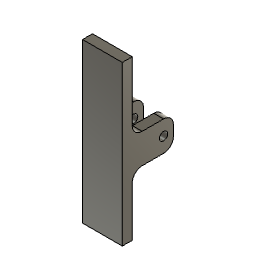
bending_tool_base v2 (Autodesk Fusion 360 design; units mm, degrees)
Autodesk Fusion 360 part; units mm, degrees
sketch "Skizze8" plane through (0, 0, 0) normal (1, 0, 0) x (0, 1, 0)
  line L0 (-6.5, 80) -> (-16.5, 80)
  line L1 (-16.5, 80) -> (-16.5, -80)
  line L2 (-16.5, -80) -> (-6.5, -80)
  line L3 (-6.5, -80) -> (-6.5, -30)
  line L4 (3.5, -20) -> (25, -20)
  line L5 (35, -10) -> (35, 0)
  line L6 (25, 10) -> (3.5, 10)
  line L7 (105.6778, -5) -> (-37.6639, -5) construction
  line L8 (25, 49.113) -> (25, -113.6091) construction
  line L9 (-6.5, 20) -> (-6.5, 80)
  arc A0 (-6.5, 20) -> (3.5, 10) centre (3.5, 20) ccw
  arc A1 (3.5, -20) -> (-6.5, -30) centre (3.5, -30) ccw
  arc A2 (35, 0) -> (25, 10) centre (25, 0) ccw
  arc A3 (25, -20) -> (35, -10) centre (25, -10) ccw
  circle A4 centre (25, -5) radius 4.15
  point P0 (-6.5, 10)
  dimension "d127" = 80
  dimension "d128" = 80
  dimension "d129" = 5
  dimension "d130" = 31.5
  dimension "d131" = 25
  dimension "d132" = 10
  dimension "d133" = 10
  dimension "d134" = 15
  dimension "d135" = 15
  dimension "d136" = 10
  dimension "d137" = 10
  dimension "d138" = 10
  dimension "d139" = 10
  dimension "d140" = 10
  dimension "d141" = 10
  dimension "d142" = 8.3
  constraint horizontal L0
  constraint perpendicular L0 L1
  constraint perpendicular L1 L2
  constraint perpendicular L2 L3
  constraint perpendicular L3 L4
  constraint perpendicular L4 L5
  constraint perpendicular L5 L6
  constraint perpendicular L1 L7
  constraint vertical L8
  constraint coincident P0 L6
  constraint coincident P0 L9
  constraint tangent L6 A0
  constraint tangent L9 A0
  constraint tangent L3 A1
  constraint tangent L4 A1
  constraint tangent L5 A2
  constraint tangent L6 A2
  constraint tangent L4 A3
  constraint tangent L5 A3
  constraint coincident L8 A4.centre
  constraint coincident L7 A4.centre
  measures "d127" distance of origin L0
  measures "d128" distance of origin L2
  measures "d129" distance of origin L7
  measures "d130" distance of L3 L8
  measures "d131" distance of origin L8
  measures "d132" distance of L1 L3
  measures "d133" distance of L5 L8
  measures "d134" distance of L4 L7
  measures "d135" distance of L6 L7
  measures "d136" distance of L0.start L1
  measures "d137" distance of L1 P0
  measures "d138" radius of A0
  measures "d139" radius of A1
  measures "d140" radius of A2
  measures "d141" radius of A3
  measures "d142" diameter of A4
extrude "Extrusion8" add sketch "Skizze8" along normal mid plane 40
sketch "Skizze9" plane through (0, 0, 0) normal (0, 0, 1) x (1, 0, 0)
  line L0 (10.1, 40) -> (-10.1, 40)
  line L1 (-10.1, 40) -> (-10.1, -6.5)
  line L2 (-10.1, -6.5) -> (10.1, -6.5)
  line L3 (10.1, -6.5) -> (10.1, 40)
  dimension "d145" = 6.5
  dimension "d146" = 40
  dimension "d147" = 10.1
  dimension "d148" = 10.1
  constraint horizontal L0
  constraint vertical L1
  constraint horizontal L2
  constraint vertical L3
  measures "d145" distance of origin L2
  measures "d146" distance of origin L0
  measures "d147" distance of origin L1
  measures "d148" distance of origin L3
extrude "Extrusion9" cut sketch "Skizze9" along normal mid plane 200
